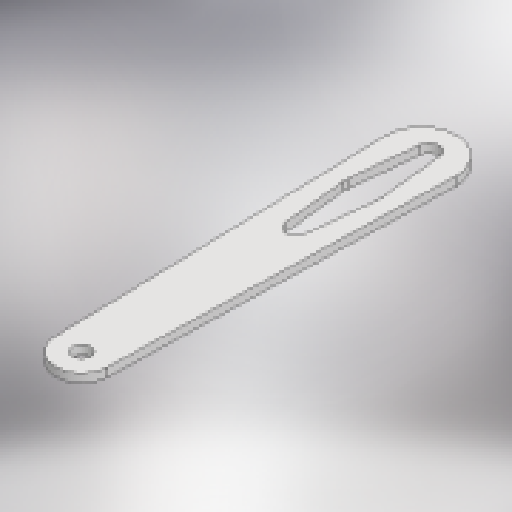
# Autodesk Inventor part: arm3
Saved by Autodesk Inventor 2024 (Build 280153000, 153)
## iProperties
Created: 2023-10-08
Part Number: arm3
Material: Generic
Document SubType Name: Modeling
Designer: byrne
Density: 1 g/cm^3
Appearance: Default
Author: byrne
Autodesk Inventor part; units mm, degrees
ref_plane "YZ Plane" through (0, 0, 0) normal (1, 0, 0) x (0, 1, 0)
ref_plane "XZ Plane" through (0, 0, 0) normal (0, 1, 0) x (-1, 0, 0)
ref_plane "XY Plane" through (0, 0, 0) normal (0, 0, 1) x (1, 0, 0)
sketch "Sketch1" plane through (0, 0, 0) normal (0, 1, 0) x (-1, 0, 0)
  arc A0 (1.4918, 12.1563) -> (-1.4918, 12.1563) centre (0, 12) ccw
  arc A1 (-1.4918, -12.1563) -> (1.4918, -12.1563) centre (0, -12) ccw
  line L0 (0, -12) -> (0, 12) construction
  line L1 (-2.735, 0.2865) -> (-1.4918, 12.1563)
  line L2 (1.4918, -12.1563) -> (2.735, -0.2865)
  line L3 (-1.4918, -12.1563) -> (-2.735, -0.2865)
  line L4 (2.735, 0.2865) -> (1.4918, 12.1563)
  arc A2 (-2.735, 0.2865) -> (-2.735, -0.2865) centre (0, 0) ccw
  arc A3 (2.735, -0.2865) -> (2.735, 0.2865) centre (0, 0) ccw
  line L5 (2.75, 0) -> (-2.75, 0) construction
  line L6 (-3.0334, -0.3177) -> (-1.7902, -12.1875)
  arc A4 (-1.7902, -12.1875) -> (1.7902, -12.1875) centre (0, -12) ccw
  line L7 (1.7902, -12.1875) -> (3.0334, -0.3177)
  arc A5 (3.0334, -0.3177) -> (3.0334, 0.3177) centre (0, 0) ccw
  line L8 (3.0334, 0.3177) -> (1.7902, 12.1875)
  arc A6 (1.7902, 12.1875) -> (-1.7902, 12.1875) centre (0, 12) ccw
  line L9 (-1.7902, 12.1875) -> (-3.0334, 0.3177)
  arc A7 (-3.0334, 0.3177) -> (-3.0334, -0.3177) centre (0, 0) ccw
  line L10 (0, -4.275) -> (0, 57.15) construction
  line L11 (-6.35, -10.625) -> (-6.35, 50.8)
  line L12 (6.35, 50.8) -> (6.35, -10.625)
  arc A8 (-6.35, -10.625) -> (6.35, -10.625) centre (0, -10.625) ccw
  arc A9 (6.35, 50.8) -> (-6.35, 50.8) centre (0, 50.8) ccw
  circle A10 centre (0, 50.8) radius 1.5875
  point P0 (0, 0)
  point P1 (0, -13.8)
  point P2 (0, -16.975)
  dimension "d5" = 3
  dimension "d6" = 3
  dimension "d7" = 24
  dimension "d8" = 5.5
  dimension "d9" = 0.3
  dimension "d13" = 50.8
  dimension "d15" = 3.175
  dimension "d17" = 3.175
  dimension "d19" = 6.35
  dimension "d20" = 6.35
  constraints: 28 end point, 26 point on circle, 12 tangent, 11 centre point, 3 coincident, 3 midpoint, 2 point on line, 2 vertical, 1 collinear, 8 other
  measures "d5" diameter of A0
  measures "d6" diameter of A1
  measures "d7" distance of L0.start L0.end
  measures "d8" distance of L5.start L5.end
  measures "d9" distance between parallel lines of L3 L6
  measures "d13" distance of point (0, 50.8) A2.centre
  measures "d15" distance of point (0, -13.8) point (0, -16.975)
  measures "d17" diameter of A10
  measures "d19" radius of A8
  measures "d20" radius of A9
extrude "Extrusion1" add sketch "Sketch1" along normal blind 1.5875 contours L11 A9 L12 A8
sketch "Sketch2" plane through (0, 1.5875, 0) normal (0, 1, 0) x (1, 0, 0)
  line L0 (6.35, -50.8) -> (6.35, 10.625) projected
  arc A0 (6.35, 10.625) -> (-6.35, 10.625) centre (0, 10.625) ccw projected
  line L1 (-6.35, 10.625) -> (-6.35, -50.8) projected
  arc A1 (-6.35, -50.8) -> (6.35, -50.8) centre (0, -50.8) ccw projected
  arc A2 (3.0334, -0.3177) -> (3.0334, 0.3177) centre (0, 0) ccw projected
  line L2 (3.0334, -0.3177) -> (1.7902, -12.1875) projected
  arc A3 (-1.7902, -12.1875) -> (1.7902, -12.1875) centre (0, -12) ccw projected
  line L3 (-1.7902, -12.1875) -> (-3.0334, -0.3177) projected
  arc A4 (-3.0334, 0.3177) -> (-3.0334, -0.3177) centre (0, 0) ccw projected
  line L4 (-3.0334, 0.3177) -> (-1.7902, 12.1875) projected
  arc A5 (1.7902, 12.1875) -> (-1.7902, 12.1875) centre (0, 12) ccw projected
  line L5 (1.7902, 12.1875) -> (3.0334, 0.3177) projected
  circle A6 centre (0, -50.8) radius 1.5875 projected
extrude "Extrusion2" add sketch "Sketch2" along normal blind 1.5875 contours A1 L1 A0 L0 | L2 A3 L3 A4 L4 A5 L5 A2
body "Solid1"
